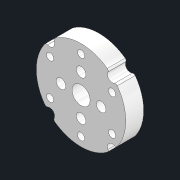
# Autodesk Inventor part: scara-base18
Saved by Autodesk Inventor 2022 (Build 260153000, 153)
## iProperties
Created: 2021-10-11
Part Number: scara-base18
Material: ABS プラスチック
Document SubType Name: Modeling
Designer: Yuta Kage
Density: 1.06 g/cm^3
Appearance: 滑らか - 白
Description: 印刷
Author: Yuta Kage
Autodesk Inventor part; units mm, degrees
ref_plane "YZ Plane" through (0, 0, 0) normal (1, 0, 0) x (0, 1, 0)
ref_plane "XZ Plane" through (0, 0, 0) normal (0, 1, 0) x (-1, 0, 0)
ref_plane "XY Plane" through (0, 0, 0) normal (0, 0, 1) x (1, 0, 0)
sketch "スケッチ1" plane through (0, 0, 0) normal (0, 0, 1) x (1, 0, 0)
  circle A0 centre (0, 0) radius 20
  dimension "d0" = 40
  constraints: 1 centre point, 1 coincident
  measures "d0" diameter of A0
extrude "押し出し1" add sketch "スケッチ1" along normal blind 8
sketch "スケッチ2" plane through (0, 0, 8) normal (0, 0, 1) x (1, 0, 0)
  circle A0 centre (0, 0) radius 16
  point P0 (0, 16)
  point P1 (-13.8564, 8)
  point P2 (-13.8564, -8)
  point P3 (0, -16)
  point P4 (13.8564, -8)
  point P5 (13.8564, 8)
  dimension "d3" = 32
  dimension "d6" = 360
  constraints: 1 coincident, 1 vertical alignment, 9 other
hole "穴1" at (0, 16, 8) at (-13.8564, 8, 8) at (-13.8564, -8, 8) at (0, -16, 8) at (13.8564, -8, 8) at (13.8564, 8, 8) direction (0, 0, -1) diameter 3.2 end through all clearance for "Socket Head Cap Screw" size "M3" standard "Ansi Metric M Profile"
sketch "スケッチ3" plane through (0, 0, 0) normal (0, 0, -1) x (-1, 0, 0)
  circle A0 centre (0, 0) radius 9
  point P0 (0, 9)
  point P1 (-9, 0)
  point P2 (0, -9)
  point P3 (9, 0)
  dimension "d15" = 18
  dimension "d18" = 360
  constraints: 1 coincident, 1 vertical alignment, 7 other
hole "穴2" at (0, 9, 0) at (9, 0, 0) at (0, -9, 0) at (-9, 0, 0) direction (0, 0, 1) diameter 4.3 end through all clearance for "Socket Head Cap Screw" size "M4" standard "Ansi Metric M Profile"
sketch "スケッチ4" plane through (0, 0, 8) normal (0, 0, 1) x (1, 0, 0)
  circle A0 centre (0, 0) radius 4.05
  dimension "d27" = 8.1
  constraints: 1 centre point, 1 coincident
  measures "d27" diameter of A0
extrude "押し出し2" cut sketch "スケッチ4" against normal blind 6
sketch "スケッチ5" plane through (0, 0, 8) normal (0, 0, 1) x (1, 0, 0)
  line L0 (-14, -14) -> (14, -14)
  line L1 (14, -14) -> (14, 14)
  line L2 (14, 14) -> (-14, 14)
  line L3 (-14, 14) -> (-14, -14)
  line L4 (-14, -14) -> (14, 14) construction
  line L5 (14, -14) -> (-14, 14) construction
  point P0 (0, 0)
  dimension "d30" = 28
  dimension "d31" = 28
  constraints: 12 end point, 2 midpoint, 2 parallel, 1 horizontal, 1 perpendicular
  measures "d30" distance of L2.end L1.end
  measures "d31" distance of L1.end L0.end
hole "穴3" at (-14, 14, 8) at (14, 14, 8) at (14, -14, 8) at (-14, -14, 8) direction (0, 0, -1) diameter 2.2 end through all counterbore diameter 4.4 counterbore depth 20 clearance for "Socket Head Cap Screw" size "M2" standard "Ansi Metric M Profile"
fillet "フィレット1" radius 1 8 edges at (-15.611, -12.5018, 4) (-12.5018, -15.611, 4) (12.5018, -15.611, 4) (15.611, -12.5018, 4) (15.611, 12.5018, 4) (12.5018, 15.611, 4) (-15.611, 12.5018, 4) (-12.5018, 15.611, 4)
